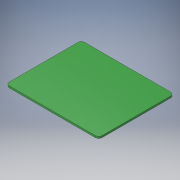
# Autodesk Inventor part: Receiver PCB
Saved by Autodesk Inventor 2017.3 (Build 213256000, 256)
## iProperties
Created: 2019-01-12
Part Number: Receiver PCB
Material: Generic
Document SubType Name: Modeling
Designer: LSabe
Density: 1 g/cm^3
Appearance: Default
Author: LSabe
Autodesk Inventor part; units mm, degrees
ref_plane "YZ Plane" through (0, 0, 0) normal (1, 0, 0) x (0, 1, 0)
ref_plane "XZ Plane" through (0, 0, 0) normal (0, 1, 0) x (-1, 0, 0)
ref_plane "XY Plane" through (0, 0, 0) normal (0, 0, 1) x (1, 0, 0)
sketch "Sketch1" plane through (0, 0, 0) normal (0, 1, 0) x (-1, 0, 0)
  line L0 (0, 0) -> (-87.7824, 0)
  line L1 (-87.7824, 0) -> (-87.7824, -71.2724)
  line L2 (-87.7824, -71.2724) -> (0, -71.2724)
  line L3 (0, -71.2724) -> (0, 0)
  dimension "d0" = 87.7824
  dimension "d1" = 71.2724
  constraints: 8 end point, 2 parallel, 1 horizontal, 1 perpendicular
  measures "d0" distance of L2.end L1.end
  measures "d1" distance of L1.end L0.end
extrude "Extrusion1" add sketch "Sketch1" along normal blind 1.778
fillet "Fillet1" radius 3.175 4 edges at (0, 0.889, 0) (0, 0.889, -71.2724) (87.7824, 0.889, -71.2724) (87.7824, 0.889, 0)
ref_plane "Work Plane1" through (43.8912, 0, -3.175) normal (1, 0, 0) x (0, 0, -1)
body "Solid1"
